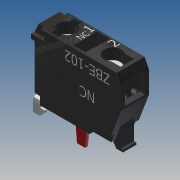
# Autodesk Inventor part: Contact NC
Saved by Autodesk Inventor 2014 (Build 180170000, 170)
## iProperties
Created: 2014-11-10
Part Number: Contact NC
Material: PPS Plastic
Document SubType Name: Modeling
Designer: David
Density: 1.637 g/cm^3
Appearance: Rubber - Black - Version 1.1
Description: CONTACT BLOCK, 1NC, 6A
Author: David
Autodesk Inventor part; units mm, degrees
ref_plane "YZ Plane" through (0, 0, 0) normal (1, 0, 0) x (0, 1, 0)
ref_plane "XZ Plane" through (0, 0, 0) normal (0, 1, 0) x (-1, 0, 0)
sketch "Sketch1" plane through (0, 0, 0) normal (0, 0, 1) x (1, 0, 0)
  line L0 (0, -3.175) -> (0, -22.0345)
  line L1 (3.175, -23.622) -> (27.2415, -23.622)
  line L2 (32.004, -10.922) -> (32.004, -3.175)
  line L3 (30.48, 0) -> (1.524, 0)
  line L4 (30.48, 0) -> (32.004, -3.175)
  line L5 (32.004, -10.922) -> (27.2415, -23.622)
  line L6 (0, -22.0345) -> (3.175, -22.0345)
  line L7 (3.175, -22.0345) -> (3.175, -23.622)
  line L8 (1.524, 0) -> (0, -3.175)
  point P0 (0, 0)
  dimension "d2" = 1.524
  dimension "d3" = 3.175
  dimension "d4" = 12.7
  dimension "d5" = 4.7625
  dimension "d6" = 32.004
  dimension "d7" = 3.175
  dimension "d8" = 1.5875
  dimension "d9" = 23.622
  constraints: 18 end point, 3 perpendicular, 2 parallel, 2 point on line, 1 equal length, 1 horizontal alignment, 1 vertical
  measures "d2" horizontal distance of L3.start L2.end
  measures "d3" vertical distance of L3.start L2.end
  measures "d4" vertical distance of L2.start L1.end
  measures "d5" horizontal distance of L2.start L1.end
  measures "d6" distance between parallel lines of L2 L0
  measures "d7" distance of L0.end L6.end
  measures "d8" distance of L1.start L6.end
  measures "d9" distance between parallel lines of L1 L3
extrude "Body" add sketch "Sketch1" along normal mid plane 9.906
sketch "Sketch2" plane through (32.004, -10.922, 4.953) normal (1, 0, 0) x (0, 0, -1)
  line L0 (1.397, 8.382) -> (8.509, 8.382)
  line L1 (8.509, 8.382) -> (8.509, 0.762)
  line L2 (8.509, 0.762) -> (1.397, 0.762)
  line L3 (1.397, 0.762) -> (1.397, 8.382)
  line L4 (4.953, -17.4244) -> (4.953, 15.6464) construction
  line L5 (0, 10.922) -> (9.906, 10.922) construction
  point P0 (4.953, 10.922)
  dimension "d12" = 2.54
  dimension "d13" = 7.62
  dimension "d14" = 7.112
  constraints: 8 end point, 2 parallel, 1 horizontal, 1 perpendicular, 1 other
  measures "d12" distance between parallel lines of L0 L5
  measures "d13" distance of L0.end L1.end
  measures "d14" distance of L0.start L0.end
extrude "Extrusion2" cut sketch "Sketch2" against normal blind 2.032
sketch "Sketch3" plane through (1.524, 0, 4.953) normal (0, 1, 0) x (1, 0, 0)
  line L0 (36.8808, 4.953) -> (-7.9248, 4.953) construction
  arc A0 (24.4451, 7.3343) -> (24.4451, 2.5718) centre (22.5425, 4.953) ccw
  line L1 (-1.524, 0) -> (-1.524, 9.906) projected
  line L2 (30.48, 8.509) -> (30.48, 9.906) projected
  line L3 (12.7635, 9.144) -> (17.2085, 9.144)
  line L4 (17.2085, 9.144) -> (17.2085, 0.762)
  line L5 (17.2085, 0.762) -> (12.7635, 0.762)
  line L6 (12.7635, 0.762) -> (12.7635, 9.144)
  line L7 (28.956, 0) -> (0, 0) projected
  line L8 (28.956, 0) -> (28.956, 9.906) projected
  line L9 (0, 9.906) -> (28.956, 9.906) projected
  line L10 (27.7654, 7.3342) -> (24.4451, 7.3343)
  line L11 (24.4451, 2.5718) -> (27.7654, 2.5718)
  line L12 (27.7654, 2.5718) -> (27.7654, 7.3342)
  line L13 (4.826, 9.144) -> (7.2072, 9.144)
  line L14 (7.2072, 0.762) -> (4.826, 0.762)
  line L15 (4.826, 0.762) -> (4.826, 2.351)
  line L16 (4.826, 7.555) -> (4.826, 9.144)
  line L17 (7.2072, 9.144) -> (7.2072, 7.8958)
  line L18 (7.2072, 2.0102) -> (7.2072, 0.762)
  arc A1 (4.826, 7.555) -> (4.826, 2.351) centre (6.4135, 4.953) ccw
  arc A2 (7.2072, 2.0102) -> (7.2072, 7.8958) centre (6.4135, 4.953) ccw
  point P0 (-1.524, 4.953)
  dimension "d17" = 6.096
  dimension "d18" = 7.9375
  dimension "d19" = 7.9375
  dimension "d20" = 8.382
  dimension "d21" = 4.445
  dimension "d22" = 14.2875
  dimension "d33" = 1.1906
  dimension "d34" = 4.7625
  dimension "d35" = 0.762
  dimension "d36" = 0.762
  dimension "d38" = 2.3813
  constraints: 26 end point, 8 parallel, 6 point on circle, 3 centre point, 3 horizontal, 3 perpendicular, 2 point on line, 2 other
  measures "d17" diameter of A0
  measures "d18" distance from line of L1 A1.centre
  measures "d19" distance from line of A0.centre L2
  measures "d20" distance of L5.end L3.start
  measures "d21" distance of L3.start L3.end
  measures "d22" distance between parallel lines of L6 L1
  measures "d33" distance between parallel lines of L12 L8
  measures "d34" distance between parallel lines of L11 L10
  measures "d35" distance between parallel lines of L13 L9
  measures "d36" distance between parallel lines of L7 L14
  measures "d38" distance of L13.start L13.end
extrude "Top" cut sketch "Sketch3" against normal blind 4.318
sketch "Sketch4" plane through (0, 0, 4.953) normal (0, 0, 1) x (1, 0, 0)
  line L0 (3.175, -23.622) -> (27.2415, -23.622) projected
  line L1 (27.2415, -23.622) -> (32.004, -10.922) projected
  line L2 (30.48, 0) -> (1.524, 0) projected
  line L3 (28.4321, -20.447) -> (23.6696, -20.447)
  line L4 (23.6696, -20.447) -> (20.8915, -23.622)
  line L5 (0, -3.175) -> (0, -22.0345) projected
  line L6 (32.004, -10.922) -> (32.004, -3.175) projected
  line L7 (0, -3.175) -> (4.7625, -3.175)
  line L8 (4.7625, -3.175) -> (4.7625, -0.762)
  line L9 (4.7625, -0.762) -> (3.556, -0.762)
  arc A0 (3.556, 0) -> (3.556, -0.762) centre (3.556, -0.381) ccw
  line L10 (1.524, 0) -> (0, -3.175) projected
  line L11 (3.556, 0) -> (1.524, 0)
  line L12 (0, -3.175) -> (1.524, 0)
  line L13 (0, -22.0345) -> (3.175, -22.0345) projected
  line L14 (3.175, -22.0345) -> (3.175, -23.622) projected
  line L15 (0, -4.7625) -> (2.3813, -4.7625)
  line L16 (2.3813, -4.7625) -> (1.5875, -12.7)
  line L17 (1.5875, -12.7) -> (3.175, -21.2408)
  line L18 (3.175, -21.2408) -> (3.175, -22.0345)
  line L19 (3.175, -22.0345) -> (0, -22.0345)
  line L20 (0, -22.0345) -> (0, -4.7625)
  point P0 (0, 0)
  dimension "d25" = 3.175
  dimension "d26" = 6.35
  dimension "d27" = 4.7625
  dimension "d42" = 0.762
  dimension "d43" = 3.175
  dimension "d44" = 4.7625
  dimension "d45" = 2.3813
  dimension "d46" = 4.7625
  dimension "d47" = 1.5875
  dimension "d48" = 12.7
  dimension "d49" = 2.3813
  constraints: 26 end point, 4 collinear, 4 perpendicular, 4 point on line, 3 tangent, 2 parallel, 2 point on circle, 1 centre point
  measures "d25" distance between parallel lines of L0 L3
  measures "d26" distance of L4.end L0.end
  measures "d27" distance of L3.start L3.end
  measures "d42" distance between parallel lines of L9 L2
  measures "d43" distance edge to line of A0 L5
  measures "d44" distance between parallel lines of L8 L5
  measures "d45" distance of L15.start L15.end
  measures "d46" distance between parallel lines of L15 L2
  measures "d47" distance from line of L5 L16.end
  measures "d48" distance from line of L2 L16.end
  measures "d49" distance from line of L17.end L0
extrude "Extrusion4" cut sketch "Sketch4" against normal blind 1.27
sketch "Sketch5" plane through (1.524, -4.318, 4.953) normal (0, 1, 0) x (1, 0, 0)
  line L0 (12.7635, 0.762) -> (12.7635, 9.144) projected
  line L1 (17.2085, 9.144) -> (17.2085, 0.762) projected
  line L2 (12.7635, 9.144) -> (17.2085, 9.144)
  line L3 (17.2085, 9.144) -> (17.2085, 7.5565)
  line L4 (17.2085, 7.5565) -> (12.7635, 7.5565)
  line L5 (12.7635, 7.5565) -> (12.7635, 9.144)
  line L6 (17.2085, 0.762) -> (12.7635, 0.762)
  line L7 (12.7635, 0.762) -> (12.7635, 2.3495)
  line L8 (12.7635, 2.3495) -> (17.2085, 2.3495)
  line L9 (17.2085, 2.3495) -> (17.2085, 0.762)
  point P0 (-1.524, 4.953)
  dimension "d30" = 1.5875
  constraints: 16 end point, 4 parallel, 2 horizontal, 2 perpendicular, 2 point on line, 1 collinear
  measures "d30" distance of L4.end L0.end
extrude "Extrusion5" cut sketch "Sketch5" against normal blind 0.762 contours L0 L8 L1 L6 | L0 L2 L1 L4
sketch "Sketch6" plane through (1.524, -4.318, 4.953) normal (0, 1, 0) x (1, 0, 0)
  arc A0 (7.2072, 2.0102) -> (7.2072, 7.8958) centre (6.4135, 4.953) ccw projected
  line L0 (24.4451, 7.3343) -> (27.7654, 7.3342) projected
  arc A1 (24.4451, 7.3343) -> (24.4451, 2.5718) centre (22.5425, 4.953) ccw projected
  line L1 (27.7654, 2.5718) -> (24.4451, 2.5718) projected
  line L2 (27.7654, 7.3342) -> (27.7654, 2.5718) projected
  circle A2 centre (6.4135, 4.953) radius 2.9618
  circle A3 centre (22.5425, 4.953) radius 2.9618
  point P0 (-1.524, 4.953)
  constraints: 2 centre point, 2 coincident, 1 equal radius
extrude "Extrusion6" add sketch "Sketch6" along normal blind 0.762 contours A2 | A3
fillet "Fillet1" radius 0.508 2 edges at (4.9757, -3.556, 0) (21.1047, -3.556, 0)
mirror "Mirror1" about plane through (0, 0, 0) normal (0, 0, 1) of "Extrusion4"
ref_plane "Work Plane1" through (16.002, -10.922, 4.953) normal (1, 0, 0) x (0, 0, -1)
mirror "Mirror2" about plane through (16.002, -10.922, 4.953) normal (1, 0, 0) of "Extrusion2"
sketch "Sketch7" plane through (0, 0, 0) normal (0, 0, 1) x (1, 0, 0)
  line L0 (0, -10.16) -> (2.032, -10.16) projected
  line L1 (0, -10.16) -> (3.175, -22.0345)
  line L2 (3.175, -22.0345) -> (0, -22.0345)
  line L3 (3.175, -21.2408) -> (3.175, -23.622) construction
  line L4 (3.175, -22.0345) -> (0, -22.0345)
  line L5 (0, -22.0345) -> (0, -10.16)
  point P0 (0, 0)
  constraints: 8 end point, 2 point on line, 1 collinear, 1 perpendicular
extrude "Extrusion7" cut sketch "Sketch7" along normal mid plane 7.112
fillet "Fillet2" radius 0.508 2 edges at (0, -22.0345, 3.6195) (0, -22.0345, -3.6195)
sketch "Sketch8" plane through (3.175, -23.622, -4.953) normal (-1, 0, 0) x (0, 0, 1)
  line L0 (9.906, 2.3813) -> (9.906, 0) projected
  line L1 (8.509, 1.5875) -> (1.397, 1.5875) projected
  line L2 (0, 0) -> (0, 2.3813) projected
  line L3 (1.27, 1.5875) -> (8.636, 1.5875)
  line L4 (9.906, 0.3175) -> (9.906, -3.302)
  line L5 (9.906, -3.302) -> (9.271, -3.302)
  line L6 (9.271, -3.302) -> (9.271, 0.3175)
  line L7 (8.636, 0.9525) -> (1.27, 0.9525)
  line L8 (0.635, 0.3175) -> (0.635, -3.302)
  line L9 (0.635, -3.302) -> (0, -3.302)
  line L10 (0, -3.302) -> (0, 0.3175)
  arc A0 (1.27, 0.9525) -> (0.635, 0.3175) centre (1.27, 0.3175) ccw
  arc A1 (9.271, 0.3175) -> (8.636, 0.9525) centre (8.636, 0.3175) ccw
  arc A2 (1.27, 1.5875) -> (0, 0.3175) centre (1.27, 0.3175) ccw
  arc A3 (9.906, 0.3175) -> (8.636, 1.5875) centre (8.636, 0.3175) ccw
  line L11 (9.906, 0) -> (0, 0) projected
  point P0 (4.953, 23.622)
  point P1 (0, 1.5875)
  point P2 (9.906, 1.5875)
  dimension "d53" = 0.635
  dimension "d54" = 0.635
  dimension "d55" = 0.635
  dimension "d56" = 1.27
  dimension "d63" = 3.302
  constraints: 16 end point, 8 point on circle, 8 tangent, 6 point on line, 4 centre point, 3 parallel, 3 perpendicular, 2 collinear, 2 equal length, 2 equal radius
  measures "d53" distance of L8.end L9.end
  measures "d54" distance between parallel lines of L7 L1
  measures "d55" radius of A0
  measures "d56" radius of A2
  measures "d63" distance between parallel lines of L5 L11
extrude "Extrusion8" add sketch "Sketch8" along normal blind 2.54 contours L0 L11 L6 A1 L7 A0 L8 L2 A2 L3 L1 A3 | L4 L5 L6 L11 | L8 L9 L10 L11
sketch "Sketch9" plane through (0, 0, 4.953) normal (0, 0, 1) x (1, 0, 0)
  line L0 (3.175, -22.0345) -> (0.635, -22.0345) projected
  line L1 (3.175, -26.924) -> (3.1496, -26.924)
  line L2 (3.1496, -26.924) -> (3.1496, -22.0345)
  line L3 (3.1496, -22.0345) -> (3.175, -22.0345)
  line L4 (3.175, -22.0345) -> (3.175, -26.924)
  point P0 (0, 0)
  dimension "d59" = 0.0254
  constraints: 8 end point, 2 parallel, 1 horizontal, 1 perpendicular, 1 point on line
  measures "d59" distance between parallel lines of L4 L2
extrude "Extrusion9" cut sketch "Sketch9" against normal through all
sketch "Sketch10" plane through (0, 0, 4.953) normal (0, 0, 1) x (1, 0, 0)
  line L0 (3.1496, -26.924) -> (3.1496, -23.3045) projected
  line L1 (0.635, -26.924) -> (0.635, -23.3045) projected
  line L2 (3.1496, -26.924) -> (0.635, -26.924) projected
  line L3 (3.1496, -26.924) -> (4.953, -25.005)
  line L4 (4.953, -25.005) -> (4.953, -24.384)
  line L5 (4.953, -24.384) -> (3.1496, -24.384)
  line L6 (3.175, -21.2408) -> (3.175, -23.622) projected
  line L7 (3.175, -23.622) -> (20.8915, -23.622) projected
  line L8 (20.8915, -23.622) -> (23.6696, -20.447) projected
  line L9 (23.6696, -20.447) -> (28.4321, -20.447) projected
  line L10 (28.4321, -20.447) -> (32.004, -10.922) projected
  line L11 (32.004, -10.922) -> (32.004, -3.175) projected
  line L12 (32.004, -3.175) -> (30.48, 0) projected
  line L13 (30.48, 0) -> (3.556, 0) projected
  arc A0 (3.556, 0) -> (3.556, -0.762) centre (3.556, -0.381) ccw projected
  line L14 (3.556, -0.762) -> (4.7625, -0.762) projected
  line L15 (4.7625, -0.762) -> (4.7625, -3.175) projected
  line L16 (4.7625, -3.175) -> (0, -3.175) projected
  line L17 (0, -3.175) -> (0, -4.7625) projected
  line L18 (0, -4.7625) -> (2.3813, -4.7625) projected
  line L19 (2.3813, -4.7625) -> (1.5875, -12.7) projected
  line L20 (1.5875, -12.7) -> (3.175, -21.2408) projected
  point P0 (0, 0)
  dimension "d62" = 4.318
  dimension "d64" = 0.762
  constraints: 6 end point, 2 perpendicular, 1 point on line
  measures "d62" distance between parallel lines of L4 L1
  measures "d64" distance between parallel lines of L5 L7
extrude "Extrusion10" add sketch "Sketch10" against normal up to surface (0.635 mm away) contours L0 L5 L4 L3
mirror "Mirror3" about plane through (0, 0, 0) normal (0, 0, 1) of "Extrusion10"
sketch "Sketch11" plane through (0, 0, 0) normal (0, 0, 1) x (1, 0, 0)
  line L0 (29.2894, 0) -> (29.2894, -4.318) construction
  line L1 (28.4321, -20.447) -> (32.004, -10.922) construction
  line L2 (29.2894, -18.161) -> (29.2894, -25.2095)
  line L3 (29.2894, -25.2095) -> (30.0831, -25.2095)
  line L4 (30.0831, -25.2095) -> (30.0831, -26.0032)
  line L5 (30.0831, -26.0032) -> (27.7019, -26.0032)
  line L6 (27.7019, -26.0032) -> (26.1144, -23.622)
  line L7 (28.4321, -20.447) -> (27.2415, -23.622) construction
  line L8 (23.6696, -20.447) -> (28.4321, -20.447) construction
  line L9 (20.8915, -23.622) -> (23.6696, -20.447) construction
  line L10 (27.2415, -23.622) -> (20.8915, -23.622) construction
  line L11 (26.1144, -23.622) -> (27.2415, -23.622)
  line L12 (27.2415, -23.622) -> (29.2894, -18.161)
  point P0 (0, 0)
  dimension "d67" = 1.5875
  dimension "d68" = 2.3813
  dimension "d69" = 0.7937
  dimension "d70" = 2.3813
  dimension "d71" = 3.175
  constraints: 14 end point, 4 collinear, 2 parallel, 2 point on line, 1 perpendicular
  measures "d67" distance between parallel lines of L3 L11
  measures "d68" distance between parallel lines of L5 L10
  measures "d69" distance of L2.end L3.end
  measures "d70" distance of L4.end L5.end
  measures "d71" distance from line of L6.end L2
extrude "Extrusion11" add sketch "Sketch11" along normal mid plane 4.699
sketch "Sketch12" plane through (3.175, -23.622, -4.953) normal (0, -1, 0) x (1, 0, 0)
  line L0 (24.0665, 8.636) -> (17.7165, 8.636) projected
  line L1 (17.7165, 1.27) -> (24.0665, 1.27) projected
  line L2 (11.4819, 8.636) -> (15.1649, 8.636)
  line L3 (15.1649, 8.636) -> (15.1649, 1.27)
  line L4 (15.1649, 1.27) -> (11.4819, 1.27)
  line L5 (11.4819, 1.27) -> (11.4819, 8.636)
  point P0 (-3.175, 4.953)
  dimension "d74" = 3.683
  constraints: 8 end point, 2 collinear, 2 parallel, 1 horizontal, 1 perpendicular
  measures "d74" distance between parallel lines of L5 L3
extrude "Extrusion12" add sketch "Sketch12" along normal blind 1.5875
sketch "Sketch13" plane through (3.175, -25.2095, -4.953) normal (0, -1, 0) x (1, 0, 0)
  line L0 (11.4819, 8.636) -> (11.4819, 1.27) projected
  line L1 (15.1649, 1.27) -> (15.1649, 8.636) projected
  line L2 (11.4819, 8.636) -> (15.1649, 8.636)
  line L3 (15.1649, 8.636) -> (15.1649, 7.62)
  line L4 (15.1649, 7.62) -> (11.4819, 7.62)
  line L5 (11.4819, 7.62) -> (11.4819, 8.636)
  line L6 (15.1649, 1.27) -> (11.4819, 1.27)
  line L7 (11.4819, 1.27) -> (11.4819, 2.286)
  line L8 (11.4819, 2.286) -> (15.1649, 2.286)
  line L9 (15.1649, 2.286) -> (15.1649, 1.27)
  point P0 (-3.175, 4.953)
  dimension "d77" = 1.016
  constraints: 16 end point, 4 parallel, 2 horizontal, 2 perpendicular, 2 point on line, 1 collinear
  measures "d77" distance of L4.end L0.start
extrude "Extrusion13" add sketch "Sketch13" along normal blind 4.7625 contours L2 L1 L4 L0 | L8 L1 L6 L0
chamfer "Chamfer1" distance 4.7625 distance2 0.3969 1 edges at (18.3399, -29.972, 3.175) measured on face at (18.3399, -24.1512, 0.889)
chamfer "Chamfer2" distance 4.7625 distance2 0.3969 1 edges at (18.3399, -29.972, -3.175) measured on face at (18.3399, -24.1512, 0.889)
chamfer "Chamfer3" distance 4.7625 distance2 0.3969 1 edges at (14.6569, -29.972, 3.175) measured on face at (14.6569, -24.1512, 0.889)
chamfer "Chamfer4" distance 4.7625 distance2 0.3969 1 edges at (14.6569, -29.972, -3.175) measured on face at (14.6569, -24.1512, -0.889)
sketch "Sketch14" plane through (30.48, 0, 4.953) normal (0, 1, 0) x (1, 0, 0)
  line L0 (-19.7612, 0.9488) -> (-19.7612, 10.0183) construction
  line L1 (-19.7612, 10.0183) -> (-15.2645, 10.0183) construction
  line L2 (-15.2645, 10.0183) -> (-15.2645, 0.9488) construction
  line L3 (-15.2645, 0.9488) -> (-19.7612, 0.9488) construction
  line L4 (-20.1291, 7.4413) -> (-20.1291, 9.7286) construction
  line L5 (-20.1291, 9.7286) -> (-17.0712, 9.7286) construction
  line L6 (-17.0712, 9.7286) -> (-17.0712, 7.4413) construction
  line L7 (-17.0712, 7.4413) -> (-20.1291, 7.4413) construction
  line L8 (-11.264, 7.4413) -> (-11.264, 9.7286) construction
  line L9 (-11.264, 9.7286) -> (-8.2061, 9.7286) construction
  line L10 (-8.2061, 9.7286) -> (-8.2061, 7.4413) construction
  line L11 (-8.2061, 7.4413) -> (-11.264, 7.4413) construction
  line L12 (-17.0712, 9.3902) -> (-17.0712, 7.9032)
  line L13 (-17.0712, 7.9032) -> (-17.3824, 7.9032)
  line L14 (-17.3824, 7.9032) -> (-17.3824, 8.4565)
  line L15 (-17.3824, 8.4565) -> (-19.4251, 8.4565)
  line L16 (-19.4251, 8.4565) -> (-19.4251, 7.9032)
  line L17 (-19.4251, 7.9032) -> (-19.7042, 7.9032)
  spline S0 degree 2 poles (-19.7042, 7.9032) (-19.7042, 8.2169) (-19.8821, 8.5133) (-20.1291, 8.5331) knots 0 0 0 1 2 2 2
  line L18 (-20.1291, 8.5331) -> (-20.1291, 8.8492)
  line L19 (-20.1291, 8.8492) -> (-17.3824, 8.8492)
  line L20 (-17.3824, 8.8492) -> (-17.3824, 9.3902)
  line L21 (-17.3824, 9.3902) -> (-17.0712, 9.3902)
  line L22 (-16.4968, 5.3716) -> (-16.4968, 5.0686)
  line L23 (-16.4968, 5.0686) -> (-18.2489, 4.1695)
  line L24 (-18.2489, 4.1695) -> (-16.4968, 4.1695)
  line L25 (-16.4968, 4.1695) -> (-16.4968, 3.9176)
  line L26 (-16.4968, 3.9176) -> (-18.5288, 3.9176)
  line L27 (-18.5288, 3.9176) -> (-18.5288, 4.3012)
  line L28 (-18.5288, 4.3012) -> (-16.92, 5.1196)
  line L29 (-16.92, 5.1196) -> (-18.5288, 5.1196)
  line L30 (-18.5288, 5.1196) -> (-18.5288, 5.3716)
  line L31 (-18.5288, 5.3716) -> (-16.4968, 5.3716)
  spline S1 degree 2 poles (-16.4606, 6.5769) (-16.4606, 6.3793) (-16.594, 6.0451) (-16.7274, 5.9232) knots 0 0 0 1 2 2 2
  spline S2 degree 2 poles (-16.7274, 5.9232) (-16.8591, 5.8014) (-17.2543, 5.668) (-17.5112, 5.668) knots 0 0 0 1 2 2 2
  spline S3 degree 2 poles (-17.5112, 5.668) (-17.7664, 5.668) (-18.1452, 5.7981) (-18.2851, 5.9216) knots 0 0 0 1 2 2 2
  spline S4 degree 2 poles (-18.2851, 5.9216) (-18.4218, 6.0434) (-18.5651, 6.376) (-18.5651, 6.5819) knots 0 0 0 1 2 2 2
  spline S5 degree 2 poles (-18.5651, 6.5819) (-18.5651, 6.684) (-18.5354, 6.8635) (-18.5124, 6.9392) knots 0 0 0 1 2 2 2
  spline S6 degree 2 poles (-18.5124, 6.9392) (-18.491, 7.0051) (-18.43, 7.1418) (-18.3938, 7.2093) knots 0 0 0 1 2 2 2
  line L32 (-18.3938, 7.2093) -> (-18.0678, 7.2093)
  line L33 (-18.0678, 7.2093) -> (-18.0678, 7.1879)
  spline S7 degree 2 poles (-18.0678, 7.1879) (-18.1007, 7.1516) (-18.1929, 7.0397) (-18.2374, 6.959) knots 0 0 0 1 2 2 2
  spline S8 degree 2 poles (-18.2374, 6.959) (-18.2802, 6.8816) (-18.3345, 6.6988) (-18.3345, 6.5802) knots 0 0 0 1 2 2 2
  spline S9 degree 2 poles (-18.3345, 6.5802) (-18.3345, 6.4501) (-18.2275, 6.218) (-18.1254, 6.1307) knots 0 0 0 1 2 2 2
  spline S10 degree 2 poles (-18.1254, 6.1307) (-18.0217, 6.0451) (-17.7071, 5.9496) (-17.5112, 5.9496) knots 0 0 0 1 2 2 2
  spline S11 degree 2 poles (-17.5112, 5.9496) (-17.3021, 5.9496) (-17.0007, 6.05) (-16.897, 6.1373) knots 0 0 0 1 2 2 2
  spline S12 degree 2 poles (-16.897, 6.1373) (-16.7965, 6.2229) (-16.6944, 6.4518) (-16.6944, 6.5802) knots 0 0 0 1 2 2 2
  spline S13 degree 2 poles (-16.6944, 6.5802) (-16.6944, 6.6971) (-16.7521, 6.8964) (-16.7949, 6.9738) knots 0 0 0 1 2 2 2
  spline S14 degree 2 poles (-16.7949, 6.9738) (-16.8377, 7.0479) (-16.9266, 7.1582) (-16.9579, 7.1895) knots 0 0 0 1 2 2 2
  line L34 (-16.9579, 7.1895) -> (-16.9579, 7.2093)
  line L35 (-16.9579, 7.2093) -> (-16.6352, 7.2093)
  spline S15 degree 2 poles (-16.6352, 7.2093) (-16.6039, 7.1418) (-16.5462, 7.0232) (-16.5199, 6.9392) knots 0 0 0 1 2 2 2
  spline S16 degree 2 poles (-16.5199, 6.9392) (-16.4903, 6.8503) (-16.4606, 6.6988) (-16.4606, 6.5769) knots 0 0 0 1 2 2 2
  line L36 (-8.1789, 9.5433) -> (-8.1789, 7.6636)
  line L37 (-8.1789, 7.6636) -> (-8.6112, 7.6636)
  spline S17 degree 2 poles (-8.6112, 7.6636) (-8.8014, 7.8662) (-9.1546, 8.2268) (-9.3448, 8.3997) knots 0 0 0 1 2 2 2
  spline S18 degree 2 poles (-9.3448, 8.3997) (-9.7276, 8.748) (-10.187, 9.0024) (-10.4316, 9.0024) knots 0 0 0 1 2 2 2
  spline S19 degree 2 poles (-10.4316, 9.0024) (-10.56, 9.0024) (-10.7527, 8.9233) (-10.8144, 8.8517) knots 0 0 0 1 2 2 2
  spline S20 degree 2 poles (-10.8144, 8.8517) (-10.8762, 8.7801) (-10.9379, 8.5924) (-10.9379, 8.4787) knots 0 0 0 1 2 2 2
  spline S21 degree 2 poles (-10.9379, 8.4787) (-10.9379, 8.3701) (-10.8836, 8.1478) (-10.8416, 8.0465) knots 0 0 0 1 2 2 2
  spline S22 degree 2 poles (-10.8416, 8.0465) (-10.807, 7.96) (-10.7082, 7.7995) (-10.6736, 7.7501) knots 0 0 0 1 2 2 2
  line L38 (-10.6736, 7.7501) -> (-10.6736, 7.7279)
  line L39 (-10.6736, 7.7279) -> (-11.1084, 7.7279)
  spline S23 degree 2 poles (-11.1084, 7.7279) (-11.1701, 7.8538) (-11.2911, 8.3058) (-11.2911, 8.5084) knots 0 0 0 1 2 2 2
  spline S24 degree 2 poles (-11.2911, 8.5084) (-11.2911, 8.9357) (-10.8391, 9.4174) (-10.4538, 9.4174) knots 0 0 0 1 2 2 2
  spline S25 degree 2 poles (-10.4538, 9.4174) (-10.2735, 9.4174) (-9.9721, 9.3334) (-9.8437, 9.2593) knots 0 0 0 1 2 2 2
  spline S26 degree 2 poles (-9.8437, 9.2593) (-9.7103, 9.1852) (-9.4485, 8.9703) (-9.3225, 8.8517) knots 0 0 0 1 2 2 2
  spline S27 degree 2 poles (-9.3225, 8.8517) (-9.1126, 8.6591) (-8.663, 8.1873) (-8.5321, 8.0465) knots 0 0 0 1 2 2 2
  line L40 (-8.5321, 8.0465) -> (-8.5321, 9.5433)
  line L41 (-8.5321, 9.5433) -> (-8.1789, 9.5433)
  point P0 (-30.48, 4.953)
  constraints: 6 other
extrude "Extrusion14" cut sketch "Sketch14" against normal blind 0.0254
sketch "Sketch15" plane through (0, 0, 4.953) normal (0, 0, 1) x (1, 0, 0)
  line L0 (32.8553, -6.0454) -> (6.9418, -6.0454) construction
  line L1 (6.9418, -6.0454) -> (6.9418, -1.1034) construction
  line L2 (6.9418, -1.1034) -> (32.8553, -1.1034) construction
  line L3 (32.8553, -1.1034) -> (32.8553, -6.0454) construction
  line L4 (32.8553, -14.3486) -> (6.9418, -14.3486) construction
  line L5 (6.9418, -14.3486) -> (6.9418, -9.4067) construction
  line L6 (6.9418, -9.4067) -> (32.8553, -9.4067) construction
  line L7 (32.8553, -9.4067) -> (32.8553, -14.3486) construction
  line L8 (25.6503, -1.9869) -> (27.8682, -1.9869)
  line L9 (27.8682, -1.9869) -> (27.8682, -2.3806)
  line L10 (27.8682, -2.3806) -> (26.1701, -4.7863)
  line L11 (26.1701, -4.7863) -> (27.791, -4.7863)
  line L12 (27.791, -4.7863) -> (27.791, -5.1619)
  line L13 (27.791, -5.1619) -> (25.6941, -5.1619)
  line L14 (25.6941, -5.1619) -> (25.6941, -4.7811)
  line L15 (25.6941, -4.7811) -> (27.4102, -2.3626)
  line L16 (27.4102, -2.3626) -> (25.6503, -2.3626)
  line L17 (25.6503, -2.3626) -> (25.6503, -1.9869)
  spline S0 degree 2 poles (23.08, -2.9621) (23.08, -2.7253) (23.2601, -2.3626) (23.4093, -2.2442) knots 0 0 0 1 2 2 2
  spline S1 degree 2 poles (23.4093, -2.2442) (23.5894, -2.1053) (23.9985, -1.9869) (24.3227, -1.9869) knots 0 0 0 1 2 2 2
  line L18 (24.3227, -1.9869) -> (25.2335, -1.9869)
  line L19 (25.2335, -1.9869) -> (25.2335, -5.1619)
  line L20 (25.2335, -5.1619) -> (24.3922, -5.1619)
  spline S2 degree 2 poles (24.3922, -5.1619) (24.0525, -5.1619) (23.7129, -5.1182) (23.5585, -5.0333) knots 0 0 0 1 2 2 2
  spline S3 degree 2 poles (23.5585, -5.0333) (23.3862, -4.9432) (23.2292, -4.6473) (23.2292, -4.4466) knots 0 0 0 1 2 2 2
  spline S4 degree 2 poles (23.2292, -4.4466) (23.2292, -4.2228) (23.4659, -3.8677) (23.6743, -3.7674) knots 0 0 0 1 2 2 2
  line L21 (23.6743, -3.7674) -> (23.6743, -3.7519)
  spline S5 degree 2 poles (23.6743, -3.7519) (23.3913, -3.6748) (23.08, -3.2657) (23.08, -2.9621) knots 0 0 0 1 2 2 2
  spline S6 degree 2 poles (23.5199, -2.944) (23.5199, -3.1241) (23.6229, -3.3557) (23.7772, -3.438) knots 0 0 0 1 2 2 2
  spline S7 degree 2 poles (23.7772, -3.438) (23.8776, -3.4895) (24.1143, -3.5204) (24.333, -3.5204) knots 0 0 0 1 2 2 2
  line L22 (24.333, -3.5204) -> (24.8116, -3.5204)
  line L23 (24.8116, -3.5204) -> (24.8116, -2.3471)
  line L24 (24.8116, -2.3471) -> (24.4694, -2.3471)
  spline S8 degree 2 poles (24.4694, -2.3471) (24.1915, -2.3471) (23.8724, -2.3986) (23.7489, -2.4809) knots 0 0 0 1 2 2 2
  spline S9 degree 2 poles (23.7489, -2.4809) (23.6306, -2.5658) (23.5199, -2.7768) (23.5199, -2.944) knots 0 0 0 1 2 2 2
  spline S10 degree 2 poles (23.6692, -4.3875) (23.6692, -4.5007) (23.7464, -4.6705) (23.8313, -4.7194) knots 0 0 0 1 2 2 2
  spline S11 degree 2 poles (23.8313, -4.7194) (23.9342, -4.776) (24.1838, -4.8017) (24.4076, -4.8017) knots 0 0 0 1 2 2 2
  line L25 (24.4076, -4.8017) -> (24.8116, -4.8017)
  line L26 (24.8116, -4.8017) -> (24.8116, -3.8729)
  line L27 (24.8116, -3.8729) -> (24.333, -3.8729)
  spline S12 degree 2 poles (24.333, -3.8729) (24.1349, -3.8729) (23.9471, -3.914) (23.8467, -3.9784) knots 0 0 0 1 2 2 2
  spline S13 degree 2 poles (23.8467, -3.9784) (23.7489, -4.0401) (23.6692, -4.2382) (23.6692, -4.3875) knots 0 0 0 1 2 2 2
  line L28 (22.6606, -1.9869) -> (22.6606, -5.1619)
  line L29 (22.6606, -5.1619) -> (20.6743, -5.1619)
  line L30 (20.6743, -5.1619) -> (20.6743, -4.7863)
  line L31 (20.6743, -4.7863) -> (22.2386, -4.7863)
  line L32 (22.2386, -4.7863) -> (22.2386, -3.9166)
  line L33 (22.2386, -3.9166) -> (20.7798, -3.9166)
  line L34 (20.7798, -3.9166) -> (20.7798, -3.541)
  line L35 (20.7798, -3.541) -> (22.2386, -3.541)
  line L36 (22.2386, -3.541) -> (22.2386, -2.3626)
  line L37 (22.2386, -2.3626) -> (20.6743, -2.3626)
  line L38 (20.6743, -2.3626) -> (20.6743, -1.9869)
  line L39 (20.6743, -1.9869) -> (22.6606, -1.9869)
  line L40 (19.1382, -3.1833) -> (20.3398, -3.1833)
  line L41 (20.3398, -3.1833) -> (20.3398, -3.5693)
  line L42 (20.3398, -3.5693) -> (19.1382, -3.5693)
  line L43 (19.1382, -3.5693) -> (19.1382, -3.1833)
  line L44 (16.9178, -1.9869) -> (18.4667, -1.9869)
  line L45 (18.4667, -1.9869) -> (18.4667, -2.3111)
  line L46 (18.4667, -2.3111) -> (17.8904, -2.3111)
  line L47 (17.8904, -2.3111) -> (17.8904, -4.4389)
  line L48 (17.8904, -4.4389) -> (18.4667, -4.4389)
  line L49 (18.4667, -4.4389) -> (18.4667, -4.7297)
  spline S14 degree 2 poles (18.4667, -4.7297) (18.1399, -4.7297) (17.8312, -4.9149) (17.8106, -5.1722) knots 0 0 0 1 2 2 2
  line L50 (17.8106, -5.1722) -> (17.4813, -5.1722)
  line L51 (17.4813, -5.1722) -> (17.4813, -2.3111)
  line L52 (17.4813, -2.3111) -> (16.9178, -2.3111)
  line L53 (16.9178, -2.3111) -> (16.9178, -1.9869)
  spline S15 degree 2 poles (14.3577, -3.5744) (14.3577, -2.7202) (14.8543, -1.92) (15.3715, -1.92) knots 0 0 0 1 2 2 2
  spline S16 degree 2 poles (15.3715, -1.92) (15.8963, -1.92) (16.3878, -2.7356) (16.3878, -3.5718) knots 0 0 0 1 2 2 2
  spline S17 degree 2 poles (16.3878, -3.5718) (16.3878, -4.4312) (15.8912, -5.2262) (15.3715, -5.2262) knots 0 0 0 1 2 2 2
  spline S18 degree 2 poles (15.3715, -5.2262) (14.8492, -5.2262) (14.3577, -4.4029) (14.3577, -3.5744) knots 0 0 0 1 2 2 2
  spline S19 degree 2 poles (14.9032, -2.607) (14.8414, -2.7639) (14.79, -3.2477) (14.79, -3.5744) knots 0 0 0 1 2 2 2
  spline S20 degree 2 poles (14.79, -3.5744) (14.79, -3.9012) (14.8414, -4.3823) (14.9058, -4.5444) knots 0 0 0 1 2 2 2
  spline S21 degree 2 poles (14.9058, -4.5444) (14.9701, -4.7065) (15.1939, -4.8737) (15.3715, -4.8737) knots 0 0 0 1 2 2 2
  spline S22 degree 2 poles (15.3715, -4.8737) (15.549, -4.8737) (15.778, -4.7065) (15.8449, -4.5393) knots 0 0 0 1 2 2 2
  spline S23 degree 2 poles (15.8449, -4.5393) (15.9092, -4.3772) (15.9555, -3.8832) (15.9555, -3.5718) knots 0 0 0 1 2 2 2
  spline S24 degree 2 poles (15.9555, -3.5718) (15.9555, -3.2374) (15.9144, -2.7897) (15.8475, -2.6147) knots 0 0 0 1 2 2 2
  spline S25 degree 2 poles (15.8475, -2.6147) (15.7857, -2.45) (15.5567, -2.2725) (15.3715, -2.2725) knots 0 0 0 1 2 2 2
  spline S26 degree 2 poles (15.3715, -2.2725) (15.1965, -2.2725) (14.9675, -2.4397) (14.9032, -2.607) knots 0 0 0 1 2 2 2
  line L54 (11.9932, -1.9869) -> (13.9512, -1.9869)
  line L55 (13.9512, -1.9869) -> (13.9512, -2.4372)
  spline S27 degree 2 poles (13.9512, -2.4372) (13.7402, -2.6353) (13.3646, -3.0032) (13.1845, -3.2013) knots 0 0 0 1 2 2 2
  spline S28 degree 2 poles (13.1845, -3.2013) (12.8217, -3.6001) (12.5567, -4.0787) (12.5567, -4.3334) knots 0 0 0 1 2 2 2
  spline S29 degree 2 poles (12.5567, -4.3334) (12.5567, -4.4672) (12.639, -4.6679) (12.7136, -4.7322) knots 0 0 0 1 2 2 2
  spline S30 degree 2 poles (12.7136, -4.7322) (12.7882, -4.7966) (12.9838, -4.8609) (13.1021, -4.8609) knots 0 0 0 1 2 2 2
  spline S31 degree 2 poles (13.1021, -4.8609) (13.2153, -4.8609) (13.4469, -4.8043) (13.5524, -4.7605) knots 0 0 0 1 2 2 2
  spline S32 degree 2 poles (13.5524, -4.7605) (13.6425, -4.7245) (13.8097, -4.6216) (13.8612, -4.5856) knots 0 0 0 1 2 2 2
  line L56 (13.8612, -4.5856) -> (13.8843, -4.5856)
  line L57 (13.8843, -4.5856) -> (13.8843, -5.0384)
  spline S33 degree 2 poles (13.8843, -5.0384) (13.7531, -5.1027) (13.2822, -5.2288) (13.0713, -5.2288) knots 0 0 0 1 2 2 2
  spline S34 degree 2 poles (13.0713, -5.2288) (12.6261, -5.2288) (12.1244, -4.758) (12.1244, -4.3566) knots 0 0 0 1 2 2 2
  spline S35 degree 2 poles (12.1244, -4.3566) (12.1244, -4.1688) (12.2119, -3.8549) (12.2891, -3.7211) knots 0 0 0 1 2 2 2
  spline S36 degree 2 poles (12.2891, -3.7211) (12.3663, -3.5821) (12.5901, -3.3094) (12.7136, -3.1782) knots 0 0 0 1 2 2 2
  spline S37 degree 2 poles (12.7136, -3.1782) (12.9143, -2.9595) (13.4057, -2.4912) (13.5524, -2.3548) knots 0 0 0 1 2 2 2
  line L58 (13.5524, -2.3548) -> (11.9932, -2.3548)
  line L59 (11.9932, -2.3548) -> (11.9932, -1.9869)
  line L60 (20.0735, -10.2902) -> (20.5469, -10.2902)
  line L61 (20.5469, -10.2902) -> (21.9517, -13.0278)
  line L62 (21.9517, -13.0278) -> (21.9517, -10.2902)
  line L63 (21.9517, -10.2902) -> (22.3454, -10.2902)
  line L64 (22.3454, -10.2902) -> (22.3454, -13.4652)
  line L65 (22.3454, -13.4652) -> (21.7459, -13.4652)
  line L66 (21.7459, -13.4652) -> (20.4672, -10.9514)
  line L67 (20.4672, -10.9514) -> (20.4672, -13.4652)
  line L68 (20.4672, -13.4652) -> (20.0735, -13.4652)
  line L69 (20.0735, -13.4652) -> (20.0735, -10.2902)
  spline S38 degree 2 poles (18.1901, -10.2336) (18.4989, -10.2336) (19.0212, -10.442) (19.2116, -10.6504) knots 0 0 0 1 2 2 2
  spline S39 degree 2 poles (19.2116, -10.6504) (19.402, -10.8562) (19.6104, -11.4737) (19.6104, -11.8751) knots 0 0 0 1 2 2 2
  spline S40 degree 2 poles (19.6104, -11.8751) (19.6104, -12.2739) (19.4071, -12.8657) (19.2141, -13.0844) knots 0 0 0 1 2 2 2
  spline S41 degree 2 poles (19.2141, -13.0844) (19.0237, -13.2979) (18.504, -13.5218) (18.1824, -13.5218) knots 0 0 0 1 2 2 2
  spline S42 degree 2 poles (18.1824, -13.5218) (18.0229, -13.5218) (17.7424, -13.4755) (17.6241, -13.4394) knots 0 0 0 1 2 2 2
  spline S43 degree 2 poles (17.6241, -13.4394) (17.5211, -13.406) (17.3076, -13.3108) (17.2021, -13.2542) knots 0 0 0 1 2 2 2
  line L70 (17.2021, -13.2542) -> (17.2021, -12.7447)
  line L71 (17.2021, -12.7447) -> (17.2356, -12.7447)
  spline S44 degree 2 poles (17.2356, -12.7447) (17.2922, -12.7962) (17.4671, -12.9403) (17.5932, -13.0098) knots 0 0 0 1 2 2 2
  spline S45 degree 2 poles (17.5932, -13.0098) (17.7141, -13.0766) (17.9997, -13.1616) (18.185, -13.1616) knots 0 0 0 1 2 2 2
  spline S46 degree 2 poles (18.185, -13.1616) (18.3882, -13.1616) (18.751, -12.9943) (18.8874, -12.8348) knots 0 0 0 1 2 2 2
  spline S47 degree 2 poles (18.8874, -12.8348) (19.0212, -12.6727) (19.1704, -12.1813) (19.1704, -11.8751) knots 0 0 0 1 2 2 2
  spline S48 degree 2 poles (19.1704, -11.8751) (19.1704, -11.5483) (19.0135, -11.0775) (18.8771, -10.9154) knots 0 0 0 1 2 2 2
  spline S49 degree 2 poles (18.8771, -10.9154) (18.7433, -10.7584) (18.3857, -10.5989) (18.185, -10.5989) knots 0 0 0 1 2 2 2
  spline S50 degree 2 poles (18.185, -10.5989) (18.0023, -10.5989) (17.691, -10.689) (17.57, -10.7559) knots 0 0 0 1 2 2 2
  spline S51 degree 2 poles (17.57, -10.7559) (17.4543, -10.8228) (17.2819, -10.9617) (17.233, -11.0106) knots 0 0 0 1 2 2 2
  line L72 (17.233, -11.0106) -> (17.2021, -11.0106)
  line L73 (17.2021, -11.0106) -> (17.2021, -10.5063)
  spline S52 degree 2 poles (17.2021, -10.5063) (17.3076, -10.4574) (17.4928, -10.3673) (17.6241, -10.3262) knots 0 0 0 1 2 2 2
  spline S53 degree 2 poles (17.6241, -10.3262) (17.763, -10.2799) (17.9997, -10.2336) (18.1901, -10.2336) knots 0 0 0 1 2 2 2
  point P0 (0, 0)
  constraints: 4 other
extrude "Extrusion15" cut sketch "Sketch15" against normal blind 0.0254
sketch "Sketch16" plane through (29.972, -10.922, 4.953) normal (1, 0, 0) x (0, 0, -1)
  line L0 (8.509, 0.762) -> (1.397, 0.762) projected
  line L1 (4.953, -25.0444) -> (4.953, 16.9164) construction
  circle A0 centre (3.175, 1.9526) radius 1.1906
  circle A1 centre (6.731, 1.9526) radius 1.1906
  point P0 (4.953, 10.922)
  dimension "d96" = 2.3813
  dimension "d99" = 3.556
  constraints: 2 centre point, 2 tangent, 1 symmetric about line
  measures "d96" diameter of A1
  measures "d99" distance of A1.centre A0.centre
extrude "Extrusion16" cut sketch "Sketch16" against normal blind 3.175
mirror "Mirror4" about plane through (16.002, -10.922, 4.953) normal (1, 0, 0) of "Extrusion16"
fillet "Fillet3" radius 0.0254 8 edges at (3.175, -0.381, 4.953) (4.1593, -0.762, 4.953) (17.018, 0, 4.953) (3.175, -0.381, -4.953) (4.1593, -0.762, -4.953) (17.018, 0, -4.953) (12.0333, -23.622, 4.953) (12.0333, -23.622, -4.953)
body "Solid1"
